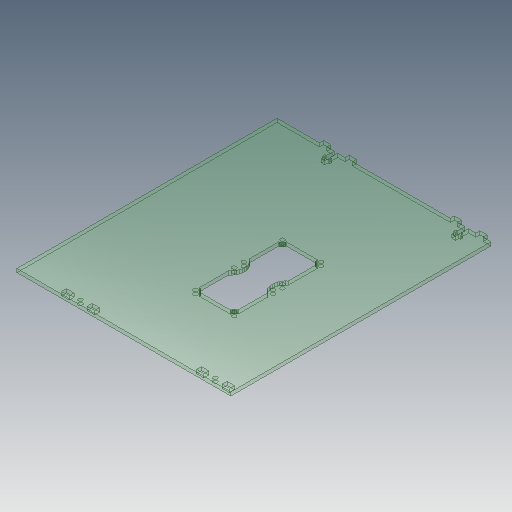
# Autodesk Inventor part: EE Top
Saved by Autodesk Inventor 2017 (Build 210142000, 142)
## iProperties
Created: 2016-07-27
Part Number: EE Top
Material: Polycarbonate, Green
Document SubType Name: Modeling
Designer: User
Density: 1.2 g/cm^3
Appearance: Polycarbonate - Clear(2)
Mass: 128.656 g
Surface Area: 752.573 cm^2
Volume: 107.213 cm^3
Author: User
Autodesk Inventor part; units mm, degrees
ref_plane "YZ Plane" through (0, 0, 0) normal (1, 0, 0) x (0, 1, 0)
ref_plane "XZ Plane" through (0, 0, 0) normal (0, 1, 0) x (-1, 0, 0)
ref_plane "XY Plane" through (0, 0, 0) normal (0, 0, 1) x (1, 0, 0)
sketch "Sketch1" plane through (0, 0, 0) normal (0, 1, 0) x (-1, 0, 0)
  line L0 (19.376, -30.1615) -> (19.376, -245.3788)
  line L1 (19.376, -245.3788) -> (25.876, -245.3788)
  line L2 (25.876, -245.3788) -> (25.876, -248.7288)
  line L3 (25.876, -248.7288) -> (31.8761, -248.7288)
  line L4 (31.8761, -248.7288) -> (31.8761, -245.3788)
  line L5 (31.8761, -245.3788) -> (37.9761, -245.3788)
  line L6 (37.9761, -245.3788) -> (37.9761, -239.3788)
  line L7 (37.9761, -239.3788) -> (36.7261, -239.3788)
  line L8 (36.7261, -239.3788) -> (36.7261, -237.3788)
  line L9 (36.7261, -237.3788) -> (37.9761, -237.3788)
  line L10 (37.9761, -237.3788) -> (37.9761, -234.7288)
  line L11 (37.9761, -234.7288) -> (40.9761, -234.7288)
  line L12 (40.9761, -234.7288) -> (40.9761, -237.3788)
  line L13 (40.9761, -237.3788) -> (42.226, -237.3788)
  line L14 (42.226, -237.3788) -> (42.226, -239.3788)
  line L15 (42.226, -239.3788) -> (40.9761, -239.3788)
  line L16 (40.9761, -239.3788) -> (40.9761, -245.3788)
  line L17 (40.9761, -245.3788) -> (47.0761, -245.3788)
  line L18 (47.0761, -245.3788) -> (47.0761, -248.7288)
  line L19 (47.0761, -248.7288) -> (53.076, -248.7288)
  line L20 (53.076, -248.7288) -> (53.076, -245.3788)
  line L21 (53.076, -245.3788) -> (53.1761, -245.3788)
  line L22 (53.1761, -245.3788) -> (134.0761, -245.3788)
  line L23 (134.0761, -245.3788) -> (134.0761, -248.7288)
  line L24 (134.0761, -248.7288) -> (140.0761, -248.7288)
  line L25 (140.0761, -248.7288) -> (140.0761, -245.3788)
  line L26 (140.0761, -245.3788) -> (146.176, -245.3788)
  line L27 (146.176, -245.3788) -> (146.176, -239.3788)
  line L28 (146.176, -239.3788) -> (144.926, -239.3788)
  line L29 (144.926, -239.3788) -> (144.926, -237.3788)
  line L30 (144.926, -237.3788) -> (146.176, -237.3788)
  line L31 (146.176, -237.3788) -> (146.176, -234.7288)
  line L32 (146.176, -234.7288) -> (149.1761, -234.7288)
  line L33 (149.1761, -234.7288) -> (149.1761, -237.3788)
  line L34 (149.1761, -237.3788) -> (150.4261, -237.3788)
  line L35 (150.4261, -237.3788) -> (150.4261, -239.3788)
  line L36 (150.4261, -239.3788) -> (149.1761, -239.3788)
  line L37 (149.1761, -239.3788) -> (149.1761, -245.3788)
  line L38 (149.1761, -245.3788) -> (155.2761, -245.3788)
  line L39 (155.2761, -245.3788) -> (155.2761, -248.7288)
  line L40 (155.2761, -248.7288) -> (161.276, -248.7288)
  line L41 (161.276, -248.7288) -> (161.276, -245.3788)
  line L42 (161.276, -245.3788) -> (161.376, -245.3788)
  line L43 (161.376, -245.3788) -> (196.376, -245.3788)
  line L44 (196.376, -245.3788) -> (196.376, -30.1615)
  line L45 (196.376, -30.1615) -> (19.376, -30.1615)
  line L46 (76.7649, -160.1938) -> (76.5951, -159.7839)
  line L47 (76.5951, -159.7839) -> (76.325, -159.4319)
  line L48 (76.325, -159.4319) -> (75.9729, -159.1617)
  line L49 (75.9729, -159.1617) -> (75.5628, -158.9919)
  line L50 (75.5628, -158.9919) -> (75.1229, -158.9339)
  line L51 (75.1229, -158.9339) -> (74.6829, -158.9919)
  line L52 (74.6829, -158.9919) -> (74.2729, -159.1617)
  line L53 (74.2729, -159.1617) -> (73.9208, -159.4319)
  line L54 (73.9208, -159.4319) -> (73.6506, -159.784)
  line L55 (73.6506, -159.784) -> (73.4808, -160.194)
  line L56 (73.4808, -160.194) -> (73.4229, -160.634)
  line L57 (73.4229, -160.634) -> (73.4808, -161.074)
  line L58 (73.4808, -161.074) -> (73.6506, -161.484)
  line L59 (73.6506, -161.484) -> (73.9208, -161.836)
  line L60 (73.9208, -161.836) -> (74.2729, -162.1062)
  line L61 (74.2729, -162.1062) -> (74.6829, -162.276)
  line L62 (74.6829, -162.276) -> (75.1229, -162.334)
  line L63 (75.1229, -162.334) -> (75.5629, -162.276)
  line L64 (75.5629, -162.276) -> (75.9729, -162.1062)
  line L65 (75.9729, -162.1062) -> (76.325, -161.836)
  line L66 (76.325, -161.836) -> (76.5951, -161.4839)
  line L67 (76.5951, -161.4839) -> (76.7649, -161.074)
  line L68 (76.7649, -161.074) -> (76.8229, -160.6339)
  line L69 (76.8229, -160.6339) -> (76.7649, -160.1938)
  line L70 (76.7642, -120.194) -> (76.5944, -119.784)
  line L71 (76.5944, -119.784) -> (76.3242, -119.4319)
  line L72 (76.3242, -119.4319) -> (75.9721, -119.1618)
  line L73 (75.9721, -119.1618) -> (75.5621, -118.992)
  line L74 (75.5621, -118.992) -> (75.1221, -118.934)
  line L75 (75.1221, -118.934) -> (74.6821, -118.992)
  line L76 (74.6821, -118.992) -> (74.2721, -119.1618)
  line L77 (74.2721, -119.1618) -> (73.9201, -119.4319)
  line L78 (73.9201, -119.4319) -> (73.6499, -119.7841)
  line L79 (73.6499, -119.7841) -> (73.48, -120.1941)
  line L80 (73.48, -120.1941) -> (73.4221, -120.6341)
  line L81 (73.4221, -120.6341) -> (73.48, -121.0741)
  line L82 (73.48, -121.0741) -> (73.6499, -121.4841)
  line L83 (73.6499, -121.4841) -> (73.92, -121.8361)
  line L84 (73.92, -121.8361) -> (74.2722, -122.1063)
  line L85 (74.2722, -122.1063) -> (74.6822, -122.2761)
  line L86 (74.6822, -122.2761) -> (75.1221, -122.3341)
  line L87 (75.1221, -122.3341) -> (75.5621, -122.2761)
  line L88 (75.5621, -122.2761) -> (75.9721, -122.1063)
  line L89 (75.9721, -122.1063) -> (76.3242, -121.8361)
  line L90 (76.3242, -121.8361) -> (76.5944, -121.484)
  line L91 (76.5944, -121.484) -> (76.7642, -121.074)
  line L92 (76.7642, -121.074) -> (76.8221, -120.634)
  line L93 (76.8221, -120.634) -> (76.7642, -120.194)
  line L94 (76.7643, -128.194) -> (76.5945, -127.784)
  line L95 (76.5945, -127.784) -> (76.3243, -127.4319)
  line L96 (76.3243, -127.4319) -> (75.9722, -127.1618)
  line L97 (75.9722, -127.1618) -> (75.5622, -126.9919)
  line L98 (75.5622, -126.9919) -> (75.1222, -126.934)
  line L99 (75.1222, -126.934) -> (74.6823, -126.992)
  line L100 (74.6823, -126.992) -> (74.2723, -127.1618)
  line L101 (74.2723, -127.1618) -> (73.9202, -127.432)
  line L102 (73.9202, -127.432) -> (73.65, -127.784)
  line L103 (73.65, -127.784) -> (73.4802, -128.194)
  line L104 (73.4802, -128.194) -> (73.4223, -128.6341)
  line L105 (73.4223, -128.6341) -> (73.4802, -129.074)
  line L106 (73.4802, -129.074) -> (73.65, -129.484)
  line L107 (73.65, -129.484) -> (73.9202, -129.8361)
  line L108 (73.9202, -129.8361) -> (74.2723, -130.1063)
  line L109 (74.2723, -130.1063) -> (74.6823, -130.2761)
  line L110 (74.6823, -130.2761) -> (75.1223, -130.3341)
  line L111 (75.1223, -130.3341) -> (75.5623, -130.2761)
  line L112 (75.5623, -130.2761) -> (75.9723, -130.1063)
  line L113 (75.9723, -130.1063) -> (76.3244, -129.8361)
  line L114 (76.3244, -129.8361) -> (76.5945, -129.484)
  line L115 (76.5945, -129.484) -> (76.7644, -129.074)
  line L116 (76.7644, -129.074) -> (76.8223, -128.6342)
  line L117 (76.8223, -128.6342) -> (76.7643, -128.194)
  line L118 (108.7657, -128.194) -> (108.5958, -127.7838)
  line L119 (108.5958, -127.7838) -> (108.3256, -127.4318)
  line L120 (108.3256, -127.4318) -> (107.9736, -127.1616)
  line L121 (107.9736, -127.1616) -> (107.5636, -126.9918)
  line L122 (107.5636, -126.9918) -> (107.1236, -126.9339)
  line L123 (107.1236, -126.9339) -> (106.6835, -126.9918)
  line L124 (106.6835, -126.9918) -> (106.2736, -127.1616)
  line L125 (106.2736, -127.1616) -> (105.9215, -127.4318)
  line L126 (105.9215, -127.4318) -> (105.6514, -127.7839)
  line L127 (105.6514, -127.7839) -> (105.4815, -128.1939)
  line L128 (105.4815, -128.1939) -> (105.4236, -128.6339)
  line L129 (105.4236, -128.6339) -> (105.4815, -129.0739)
  line L130 (105.4815, -129.0739) -> (105.6514, -129.4839)
  line L131 (105.6514, -129.4839) -> (105.9215, -129.8359)
  line L132 (105.9215, -129.8359) -> (106.2736, -130.1061)
  line L133 (106.2736, -130.1061) -> (106.6836, -130.2759)
  line L134 (106.6836, -130.2759) -> (107.1236, -130.3339)
  line L135 (107.1236, -130.3339) -> (107.5636, -130.2759)
  line L136 (107.5636, -130.2759) -> (107.9736, -130.1061)
  line L137 (107.9736, -130.1061) -> (108.3257, -129.8359)
  line L138 (108.3257, -129.8359) -> (108.5958, -129.4838)
  line L139 (108.5958, -129.4838) -> (108.7657, -129.0738)
  line L140 (108.7657, -129.0738) -> (108.8236, -128.6339)
  line L141 (108.8236, -128.6339) -> (108.7657, -128.194)
  line L142 (108.7648, -120.1938) -> (108.5951, -119.784)
  line L143 (108.5951, -119.784) -> (108.3249, -119.4319)
  line L144 (108.3249, -119.4319) -> (107.9728, -119.1617)
  line L145 (107.9728, -119.1617) -> (107.5628, -118.9919)
  line L146 (107.5628, -118.9919) -> (107.1228, -118.934)
  line L147 (107.1228, -118.934) -> (106.6828, -118.9919)
  line L148 (106.6828, -118.9919) -> (106.2728, -119.1617)
  line L149 (106.2728, -119.1617) -> (105.9207, -119.4319)
  line L150 (105.9207, -119.4319) -> (105.6506, -119.784)
  line L151 (105.6506, -119.784) -> (105.4807, -120.194)
  line L152 (105.4807, -120.194) -> (105.4228, -120.634)
  line L153 (105.4228, -120.634) -> (105.4808, -121.074)
  line L154 (105.4808, -121.074) -> (105.6506, -121.484)
  line L155 (105.6506, -121.484) -> (105.9208, -121.8361)
  line L156 (105.9208, -121.8361) -> (106.2728, -122.1062)
  line L157 (106.2728, -122.1062) -> (106.6828, -122.276)
  line L158 (106.6828, -122.276) -> (107.1229, -122.334)
  line L159 (107.1229, -122.334) -> (107.5628, -122.276)
  line L160 (107.5628, -122.276) -> (107.9728, -122.1062)
  line L161 (107.9728, -122.1062) -> (108.3249, -121.836)
  line L162 (108.3249, -121.836) -> (108.5951, -121.484)
  line L163 (108.5951, -121.484) -> (108.7649, -121.0739)
  line L164 (108.7649, -121.0739) -> (108.8228, -120.6341)
  line L165 (108.8228, -120.6341) -> (108.7648, -120.1938)
  line L166 (108.7648, -160.1937) -> (108.5951, -159.784)
  line L167 (108.5951, -159.784) -> (108.3249, -159.4319)
  line L168 (108.3249, -159.4319) -> (107.9728, -159.1617)
  line L169 (107.9728, -159.1617) -> (107.5628, -158.9919)
  line L170 (107.5628, -158.9919) -> (107.1228, -158.934)
  line L171 (107.1228, -158.934) -> (106.6828, -158.9919)
  line L172 (106.6828, -158.9919) -> (106.2728, -159.1617)
  line L173 (106.2728, -159.1617) -> (105.9207, -159.4319)
  line L174 (105.9207, -159.4319) -> (105.6506, -159.784)
  line L175 (105.6506, -159.784) -> (105.4807, -160.194)
  line L176 (105.4807, -160.194) -> (105.4228, -160.634)
  line L177 (105.4228, -160.634) -> (105.4808, -161.074)
  line L178 (105.4808, -161.074) -> (105.6506, -161.484)
  line L179 (105.6506, -161.484) -> (105.9208, -161.8361)
  line L180 (105.9208, -161.8361) -> (106.2728, -162.1062)
  line L181 (106.2728, -162.1062) -> (106.6828, -162.276)
  line L182 (106.6828, -162.276) -> (107.1228, -162.334)
  line L183 (107.1228, -162.334) -> (107.5628, -162.276)
  line L184 (107.5628, -162.276) -> (107.9728, -162.1062)
  line L185 (107.9728, -162.1062) -> (108.3249, -161.836)
  line L186 (108.3249, -161.836) -> (108.595, -161.4839)
  line L187 (108.595, -161.4839) -> (108.7649, -161.0739)
  line L188 (108.7649, -161.0739) -> (108.8228, -160.6341)
  line L189 (108.8228, -160.6341) -> (108.7648, -160.1937)
  line L190 (149.2477, -33.6616) -> (149.1238, -33.2802)
  line L191 (149.1238, -33.2802) -> (148.9088, -32.9416)
  line L192 (148.9088, -32.9416) -> (148.6165, -32.667)
  line L193 (148.6165, -32.667) -> (148.2651, -32.4738)
  line L194 (148.2651, -32.4738) -> (147.8766, -32.3741)
  line L195 (147.8766, -32.3741) -> (147.4755, -32.3741)
  line L196 (147.4755, -32.3741) -> (147.087, -32.4738)
  line L197 (147.087, -32.4738) -> (146.7356, -32.667)
  line L198 (146.7356, -32.667) -> (146.4432, -32.9416)
  line L199 (146.4432, -32.9416) -> (146.2283, -33.2802)
  line L200 (146.2283, -33.2802) -> (146.1044, -33.6616)
  line L201 (146.1044, -33.6616) -> (146.0792, -34.0619)
  line L202 (146.0792, -34.0619) -> (146.1543, -34.4559)
  line L203 (146.1543, -34.4559) -> (146.3251, -34.8188)
  line L204 (146.3251, -34.8188) -> (146.5807, -35.1278)
  line L205 (146.5807, -35.1278) -> (146.9052, -35.3635)
  line L206 (146.9052, -35.3635) -> (147.2781, -35.5112)
  line L207 (147.2781, -35.5112) -> (147.676, -35.5615)
  line L208 (147.676, -35.5615) -> (148.0739, -35.5112)
  line L209 (148.0739, -35.5112) -> (148.4468, -35.3636)
  line L210 (148.4468, -35.3636) -> (148.7713, -35.1278)
  line L211 (148.7713, -35.1278) -> (149.0269, -34.8188)
  line L212 (149.0269, -34.8188) -> (149.1977, -34.4559)
  line L213 (149.1977, -34.4559) -> (149.2729, -34.0619)
  line L214 (149.2729, -34.0619) -> (149.2477, -33.6616)
  line L215 (155.176, -32.0615) -> (155.176, -36.1614)
  line L216 (155.176, -36.1614) -> (161.376, -36.1614)
  line L217 (161.376, -36.1614) -> (161.376, -32.0615)
  line L218 (161.376, -32.0615) -> (155.176, -32.0615)
  line L219 (37.6477, -33.6616) -> (37.5238, -33.2802)
  line L220 (37.5238, -33.2802) -> (37.3089, -32.9416)
  line L221 (37.3089, -32.9416) -> (37.0165, -32.667)
  line L222 (37.0165, -32.667) -> (36.6651, -32.4738)
  line L223 (36.6651, -32.4738) -> (36.2766, -32.3741)
  line L224 (36.2766, -32.3741) -> (35.8755, -32.3741)
  line L225 (35.8755, -32.3741) -> (35.487, -32.4738)
  line L226 (35.487, -32.4738) -> (35.1356, -32.667)
  line L227 (35.1356, -32.667) -> (34.8432, -32.9416)
  line L228 (34.8432, -32.9416) -> (34.6283, -33.2802)
  line L229 (34.6283, -33.2802) -> (34.5044, -33.6616)
  line L230 (34.5044, -33.6616) -> (34.4792, -34.0619)
  line L231 (34.4792, -34.0619) -> (34.5543, -34.4559)
  line L232 (34.5543, -34.4559) -> (34.7251, -34.8188)
  line L233 (34.7251, -34.8188) -> (34.9808, -35.1278)
  line L234 (34.9808, -35.1278) -> (35.3052, -35.3636)
  line L235 (35.3052, -35.3636) -> (35.6781, -35.5112)
  line L236 (35.6781, -35.5112) -> (36.076, -35.5615)
  line L237 (36.076, -35.5615) -> (36.4739, -35.5112)
  line L238 (36.4739, -35.5112) -> (36.8469, -35.3636)
  line L239 (36.8469, -35.3636) -> (37.1713, -35.1278)
  line L240 (37.1713, -35.1278) -> (37.427, -34.8188)
  line L241 (37.427, -34.8188) -> (37.5977, -34.4559)
  line L242 (37.5977, -34.4559) -> (37.6729, -34.0619)
  line L243 (37.6729, -34.0619) -> (37.6477, -33.6616)
  line L244 (22.376, -32.0615) -> (22.376, -36.1614)
  line L245 (22.376, -36.1614) -> (28.576, -36.1614)
  line L246 (28.576, -36.1614) -> (28.576, -32.0615)
  line L247 (28.576, -32.0615) -> (22.376, -32.0615)
  line L248 (76.7631, -88.1941) -> (76.5933, -87.7842)
  line L249 (76.5933, -87.7842) -> (76.3232, -87.4321)
  line L250 (76.3232, -87.4321) -> (75.9711, -87.162)
  line L251 (75.9711, -87.162) -> (75.5611, -86.9921)
  line L252 (75.5611, -86.9921) -> (75.1211, -86.9342)
  line L253 (75.1211, -86.9342) -> (74.6811, -86.9921)
  line L254 (74.6811, -86.9921) -> (74.2711, -87.162)
  line L255 (74.2711, -87.162) -> (73.919, -87.4321)
  line L256 (73.919, -87.4321) -> (73.6489, -87.7842)
  line L257 (73.6489, -87.7842) -> (73.479, -88.1942)
  line L258 (73.479, -88.1942) -> (73.4211, -88.6342)
  line L259 (73.4211, -88.6342) -> (73.479, -89.0742)
  line L260 (73.479, -89.0742) -> (73.6489, -89.4842)
  line L261 (73.6489, -89.4842) -> (73.919, -89.8363)
  line L262 (73.919, -89.8363) -> (74.2711, -90.1064)
  line L263 (74.2711, -90.1064) -> (74.6811, -90.2763)
  line L264 (74.6811, -90.2763) -> (75.1211, -90.3342)
  line L265 (75.1211, -90.3342) -> (75.5611, -90.2763)
  line L266 (75.5611, -90.2763) -> (75.9711, -90.1064)
  line L267 (75.9711, -90.1064) -> (76.3232, -89.8363)
  line L268 (76.3232, -89.8363) -> (76.5933, -89.4842)
  line L269 (76.5933, -89.4842) -> (76.7632, -89.0742)
  line L270 (76.7632, -89.0742) -> (76.8211, -88.6342)
  line L271 (76.8211, -88.6342) -> (76.7631, -88.1941)
  line L272 (43.576, -32.0615) -> (43.576, -36.1614)
  line L273 (43.576, -36.1614) -> (49.7761, -36.1614)
  line L274 (49.7761, -36.1614) -> (49.7761, -32.0615)
  line L275 (49.7761, -32.0615) -> (43.576, -32.0615)
  line L276 (103.3316, -121.3347) -> (103.9565, -119.7817)
  line L277 (103.9565, -119.7817) -> (104.8108, -118.342)
  line L278 (104.8108, -118.342) -> (105.8745, -117.0494)
  line L279 (105.8745, -117.0494) -> (107.1228, -115.934)
  line L280 (107.1228, -115.934) -> (107.1228, -91.834)
  line L281 (107.1228, -91.834) -> (106.7272, -91.7535)
  line L282 (106.7272, -91.7535) -> (106.3423, -91.6314)
  line L283 (106.3423, -91.6314) -> (105.9725, -91.4692)
  line L284 (105.9725, -91.4692) -> (105.622, -91.2688)
  line L285 (105.622, -91.2688) -> (105.2948, -91.0322)
  line L286 (105.2948, -91.0322) -> (104.9946, -90.7622)
  line L287 (104.9946, -90.7622) -> (104.7246, -90.462)
  line L288 (104.7246, -90.462) -> (104.488, -90.1347)
  line L289 (104.488, -90.1347) -> (104.2876, -89.7843)
  line L290 (104.2876, -89.7843) -> (104.1254, -89.4145)
  line L291 (104.1254, -89.4145) -> (104.0033, -89.0296)
  line L292 (104.0033, -89.0296) -> (103.9228, -88.634)
  line L293 (103.9228, -88.634) -> (78.3228, -88.634)
  line L294 (78.3228, -88.634) -> (78.2515, -89.0338)
  line L295 (78.2515, -89.0338) -> (78.1364, -89.4233)
  line L296 (78.1364, -89.4233) -> (77.979, -89.7977)
  line L297 (77.979, -89.7977) -> (77.7813, -90.1524)
  line L298 (77.7813, -90.1524) -> (77.5455, -90.4832)
  line L299 (77.5455, -90.4832) -> (77.2746, -90.7858)
  line L300 (77.2746, -90.7858) -> (76.972, -91.0566)
  line L301 (76.972, -91.0566) -> (76.6413, -91.2924)
  line L302 (76.6413, -91.2924) -> (76.2866, -91.4902)
  line L303 (76.2866, -91.4902) -> (75.9122, -91.6476)
  line L304 (75.9122, -91.6476) -> (75.5227, -91.7626)
  line L305 (75.5227, -91.7626) -> (75.1228, -91.834)
  line L306 (75.1228, -91.834) -> (75.1228, -115.934)
  line L307 (75.1228, -115.934) -> (76.3711, -117.0494)
  line L308 (76.3711, -117.0494) -> (77.4349, -118.342)
  line L309 (77.4349, -118.342) -> (78.2891, -119.7817)
  line L310 (78.2891, -119.7817) -> (78.914, -121.3347)
  line L311 (78.914, -121.3347) -> (79.2949, -122.9648)
  line L312 (79.2949, -122.9648) -> (79.4228, -124.634)
  line L313 (79.4228, -124.634) -> (79.2949, -126.3031)
  line L314 (79.2949, -126.3031) -> (78.914, -127.9333)
  line L315 (78.914, -127.9333) -> (78.2891, -129.4863)
  line L316 (78.2891, -129.4863) -> (77.4349, -130.9259)
  line L317 (77.4349, -130.9259) -> (76.3711, -132.2186)
  line L318 (76.3711, -132.2186) -> (75.1228, -133.334)
  line L319 (75.1228, -133.334) -> (75.1228, -157.434)
  line L320 (75.1228, -157.434) -> (75.5524, -157.4264)
  line L321 (75.5524, -157.4264) -> (75.9786, -157.4813)
  line L322 (75.9786, -157.4813) -> (76.3922, -157.5977)
  line L323 (76.3922, -157.5977) -> (76.7845, -157.7731)
  line L324 (76.7845, -157.7731) -> (77.1471, -158.0036)
  line L325 (77.1471, -158.0036) -> (77.4723, -158.2845)
  line L326 (77.4723, -158.2845) -> (77.7532, -158.6097)
  line L327 (77.7532, -158.6097) -> (77.9837, -158.9723)
  line L328 (77.9837, -158.9723) -> (78.1591, -159.3646)
  line L329 (78.1591, -159.3646) -> (78.2755, -159.7782)
  line L330 (78.2755, -159.7782) -> (78.3304, -160.2043)
  line L331 (78.3304, -160.2043) -> (78.3228, -160.634)
  line L332 (78.3228, -160.634) -> (103.9228, -160.634)
  line L333 (103.9228, -160.634) -> (104.0073, -160.2402)
  line L334 (104.0073, -160.2402) -> (104.1324, -159.8573)
  line L335 (104.1324, -159.8573) -> (104.2966, -159.4896)
  line L336 (104.2966, -159.4896) -> (104.4983, -159.1409)
  line L337 (104.4983, -159.1409) -> (104.7352, -158.8152)
  line L338 (104.7352, -158.8152) -> (105.0048, -158.516)
  line L339 (105.0048, -158.516) -> (105.3041, -158.2464)
  line L340 (105.3041, -158.2464) -> (105.6298, -158.0095)
  line L341 (105.6298, -158.0095) -> (105.9784, -157.8078)
  line L342 (105.9784, -157.8078) -> (106.3462, -157.6435)
  line L343 (106.3462, -157.6435) -> (106.729, -157.5185)
  line L344 (106.729, -157.5185) -> (107.1228, -157.434)
  line L345 (107.1228, -157.434) -> (107.1228, -133.334)
  line L346 (107.1228, -133.334) -> (105.8745, -132.2186)
  line L347 (105.8745, -132.2186) -> (104.8108, -130.9259)
  line L348 (104.8108, -130.9259) -> (103.9565, -129.4863)
  line L349 (103.9565, -129.4863) -> (103.3316, -127.9333)
  line L350 (103.3316, -127.9333) -> (102.9508, -126.3031)
  line L351 (102.9508, -126.3031) -> (102.8228, -124.634)
  line L352 (102.8228, -124.634) -> (102.9508, -122.9648)
  line L353 (102.9508, -122.9648) -> (103.3316, -121.3347)
  line L354 (108.7664, -88.1938) -> (108.5965, -87.7838)
  line L355 (108.5965, -87.7838) -> (108.3264, -87.4317)
  line L356 (108.3264, -87.4317) -> (107.9743, -87.1615)
  line L357 (107.9743, -87.1615) -> (107.5643, -86.9917)
  line L358 (107.5643, -86.9917) -> (107.1243, -86.9338)
  line L359 (107.1243, -86.9338) -> (106.6843, -86.9917)
  line L360 (106.6843, -86.9917) -> (106.2743, -87.1616)
  line L361 (106.2743, -87.1616) -> (105.9222, -87.4317)
  line L362 (105.9222, -87.4317) -> (105.6521, -87.7838)
  line L363 (105.6521, -87.7838) -> (105.4823, -88.1938)
  line L364 (105.4823, -88.1938) -> (105.4243, -88.6338)
  line L365 (105.4243, -88.6338) -> (105.4823, -89.0738)
  line L366 (105.4823, -89.0738) -> (105.6521, -89.4838)
  line L367 (105.6521, -89.4838) -> (105.9223, -89.8359)
  line L368 (105.9223, -89.8359) -> (106.2744, -90.106)
  line L369 (106.2744, -90.106) -> (106.6843, -90.2758)
  line L370 (106.6843, -90.2758) -> (107.1244, -90.3338)
  line L371 (107.1244, -90.3338) -> (107.5643, -90.2758)
  line L372 (107.5643, -90.2758) -> (107.9743, -90.106)
  line L373 (107.9743, -90.106) -> (108.3264, -89.8358)
  line L374 (108.3264, -89.8358) -> (108.5965, -89.4838)
  line L375 (108.5965, -89.4838) -> (108.7664, -89.0738)
  line L376 (108.7664, -89.0738) -> (108.8243, -88.6336)
  line L377 (108.8243, -88.6336) -> (108.7664, -88.1938)
  line L378 (133.976, -32.0615) -> (133.976, -36.1614)
  line L379 (133.976, -36.1614) -> (140.176, -36.1614)
  line L380 (140.176, -36.1614) -> (140.176, -32.0615)
  line L381 (140.176, -32.0615) -> (133.976, -32.0615)
  constraints: 764 end point, 181 parallel, 106 perpendicular, 3 collinear
extrude "Extrusion1" add sketch "Sketch1" along normal blind 3
sketch "Sketch2" plane through (0, 3, 0) normal (0, 1, 0) x (1, 0, 0)
  line L0 (-103.3316, 121.3347) -> (-102.9508, 122.9648) projected
  line L1 (-102.9508, 122.9648) -> (-102.8228, 124.634) projected
  line L2 (-102.8228, 124.634) -> (-102.9508, 126.3031) projected
  line L3 (-102.9508, 126.3031) -> (-103.3316, 127.9333) projected
  line L4 (-103.3316, 127.9333) -> (-103.9565, 129.4863) projected
  line L5 (-103.9565, 129.4863) -> (-104.8108, 130.9259) projected
  line L6 (-104.8108, 130.9259) -> (-105.8745, 132.2186) projected
  line L7 (-105.8745, 132.2186) -> (-107.1228, 133.334) projected
  line L8 (-107.1228, 133.334) -> (-107.1228, 157.434) projected
  line L9 (-107.1228, 157.434) -> (-106.729, 157.5185) projected
  line L10 (-106.729, 157.5185) -> (-106.3462, 157.6435) projected
  line L11 (-106.3462, 157.6435) -> (-105.9784, 157.8078) projected
  line L12 (-105.9784, 157.8078) -> (-105.6298, 158.0095) projected
  line L13 (-105.6298, 158.0095) -> (-105.3041, 158.2464) projected
  line L14 (-105.3041, 158.2464) -> (-105.0048, 158.516) projected
  line L15 (-105.0048, 158.516) -> (-104.7352, 158.8152) projected
  line L16 (-104.7352, 158.8152) -> (-104.4983, 159.1409) projected
  line L17 (-104.4983, 159.1409) -> (-104.2966, 159.4896) projected
  line L18 (-104.2966, 159.4896) -> (-104.1324, 159.8573) projected
  line L19 (-104.1324, 159.8573) -> (-104.0073, 160.2402) projected
  line L20 (-104.0073, 160.2402) -> (-103.9228, 160.634) projected
  line L21 (-103.9228, 160.634) -> (-78.3228, 160.634) projected
  line L22 (-78.3228, 160.634) -> (-78.3304, 160.2043) projected
  line L23 (-78.3304, 160.2043) -> (-78.2755, 159.7782) projected
  line L24 (-78.2755, 159.7782) -> (-78.1591, 159.3646) projected
  line L25 (-78.1591, 159.3646) -> (-77.9837, 158.9723) projected
  line L26 (-77.9837, 158.9723) -> (-77.7532, 158.6097) projected
  line L27 (-77.7532, 158.6097) -> (-77.4723, 158.2845) projected
  line L28 (-77.4723, 158.2845) -> (-77.1471, 158.0036) projected
  line L29 (-77.1471, 158.0036) -> (-76.7845, 157.7731) projected
  line L30 (-76.7845, 157.7731) -> (-76.3922, 157.5977) projected
  line L31 (-76.3922, 157.5977) -> (-75.9786, 157.4813) projected
  line L32 (-75.9786, 157.4813) -> (-75.5524, 157.4264) projected
  line L33 (-75.5524, 157.4264) -> (-75.1228, 157.434) projected
  line L34 (-75.1228, 157.434) -> (-75.1228, 133.334) projected
  line L35 (-75.1228, 133.334) -> (-76.3711, 132.2186) projected
  line L36 (-76.3711, 132.2186) -> (-77.4349, 130.9259) projected
  line L37 (-77.4349, 130.9259) -> (-78.2891, 129.4863) projected
  line L38 (-78.2891, 129.4863) -> (-78.914, 127.9333) projected
  line L39 (-78.914, 127.9333) -> (-79.2949, 126.3031) projected
  line L40 (-79.2949, 126.3031) -> (-79.4228, 124.634) projected
  line L41 (-79.4228, 124.634) -> (-79.2949, 122.9648) projected
  line L42 (-79.2949, 122.9648) -> (-78.914, 121.3347) projected
  line L43 (-78.914, 121.3347) -> (-78.2891, 119.7817) projected
  line L44 (-78.2891, 119.7817) -> (-77.4349, 118.342) projected
  line L45 (-77.4349, 118.342) -> (-76.3711, 117.0494) projected
  line L46 (-76.3711, 117.0494) -> (-75.1228, 115.934) projected
  line L47 (-75.1228, 115.934) -> (-75.1228, 91.834) projected
  line L48 (-75.1228, 91.834) -> (-75.5227, 91.7626) projected
  line L49 (-75.5227, 91.7626) -> (-75.9122, 91.6476) projected
  line L50 (-75.9122, 91.6476) -> (-76.2866, 91.4902) projected
  line L51 (-76.2866, 91.4902) -> (-76.6413, 91.2924) projected
  line L52 (-76.6413, 91.2924) -> (-76.972, 91.0566) projected
  line L53 (-76.972, 91.0566) -> (-77.2746, 90.7858) projected
  line L54 (-77.2746, 90.7858) -> (-77.5455, 90.4832) projected
  line L55 (-77.5455, 90.4832) -> (-77.7813, 90.1524) projected
  line L56 (-77.7813, 90.1524) -> (-77.979, 89.7977) projected
  line L57 (-77.979, 89.7977) -> (-78.1364, 89.4233) projected
  line L58 (-78.1364, 89.4233) -> (-78.2515, 89.0338) projected
  line L59 (-78.2515, 89.0338) -> (-78.3228, 88.634) projected
  line L60 (-78.3228, 88.634) -> (-103.9228, 88.634) projected
  line L61 (-103.9228, 88.634) -> (-104.0033, 89.0296) projected
  line L62 (-104.0033, 89.0296) -> (-104.1254, 89.4145) projected
  line L63 (-104.1254, 89.4145) -> (-104.2876, 89.7843) projected
  line L64 (-104.2876, 89.7843) -> (-104.488, 90.1347) projected
  line L65 (-104.488, 90.1347) -> (-104.7246, 90.462) projected
  line L66 (-104.7246, 90.462) -> (-104.9946, 90.7622) projected
  line L67 (-104.9946, 90.7622) -> (-105.2948, 91.0322) projected
  line L68 (-105.2948, 91.0322) -> (-105.622, 91.2688) projected
  line L69 (-105.622, 91.2688) -> (-105.9725, 91.4692) projected
  line L70 (-105.9725, 91.4692) -> (-106.3423, 91.6314) projected
  line L71 (-106.3423, 91.6314) -> (-106.7272, 91.7535) projected
  line L72 (-106.7272, 91.7535) -> (-107.1228, 91.834) projected
  line L73 (-107.1228, 91.834) -> (-107.1228, 115.934) projected
  line L74 (-107.1228, 115.934) -> (-105.8745, 117.0494) projected
  line L75 (-105.8745, 117.0494) -> (-104.8108, 118.342) projected
  line L76 (-104.8108, 118.342) -> (-103.9565, 119.7817) projected
  line L77 (-103.9565, 119.7817) -> (-103.3316, 121.3347) projected
  line L78 (-155.176, 32.0615) -> (-161.376, 32.0615) projected
  line L79 (-161.376, 32.0615) -> (-161.376, 36.1614) projected
  line L80 (-161.376, 36.1614) -> (-155.176, 36.1614) projected
  line L81 (-155.176, 36.1614) -> (-155.176, 32.0615) projected
  line L82 (-43.576, 32.0615) -> (-49.7761, 32.0615) projected
  line L83 (-49.7761, 32.0615) -> (-49.7761, 36.1614) projected
  line L84 (-49.7761, 36.1614) -> (-43.576, 36.1614) projected
  line L85 (-43.576, 36.1614) -> (-43.576, 32.0615) projected
  line L86 (-133.976, 32.0615) -> (-140.176, 32.0615) projected
  line L87 (-140.176, 32.0615) -> (-140.176, 36.1614) projected
  line L88 (-140.176, 36.1614) -> (-133.976, 36.1614) projected
  line L89 (-133.976, 36.1614) -> (-133.976, 32.0615) projected
  line L90 (-22.376, 32.0615) -> (-28.576, 32.0615) projected
  line L91 (-28.576, 32.0615) -> (-28.576, 36.1614) projected
  line L92 (-28.576, 36.1614) -> (-22.376, 36.1614) projected
  line L93 (-22.376, 36.1614) -> (-22.376, 32.0615) projected
  line L94 (-76.7642, 120.194) -> (-76.8221, 120.634) projected
  line L95 (-76.8221, 120.634) -> (-76.7642, 121.074) projected
  line L96 (-76.7642, 121.074) -> (-76.5944, 121.484) projected
  line L97 (-76.5944, 121.484) -> (-76.3242, 121.8361) projected
  line L98 (-76.3242, 121.8361) -> (-75.9721, 122.1063) projected
  line L99 (-75.9721, 122.1063) -> (-75.5621, 122.2761) projected
  line L100 (-75.5621, 122.2761) -> (-75.1221, 122.3341) projected
  line L101 (-75.1221, 122.3341) -> (-74.6822, 122.2761) projected
  line L102 (-74.6822, 122.2761) -> (-74.2722, 122.1063) projected
  line L103 (-74.2722, 122.1063) -> (-73.92, 121.8361) projected
  line L104 (-73.92, 121.8361) -> (-73.6499, 121.4841) projected
  line L105 (-73.6499, 121.4841) -> (-73.48, 121.0741) projected
  line L106 (-73.48, 121.0741) -> (-73.4221, 120.6341) projected
  line L107 (-73.4221, 120.6341) -> (-73.48, 120.1941) projected
  line L108 (-73.48, 120.1941) -> (-73.6499, 119.7841) projected
  line L109 (-73.6499, 119.7841) -> (-73.9201, 119.4319) projected
  line L110 (-73.9201, 119.4319) -> (-74.2721, 119.1618) projected
  line L111 (-74.2721, 119.1618) -> (-74.6821, 118.992) projected
  line L112 (-74.6821, 118.992) -> (-75.1221, 118.934) projected
  line L113 (-75.1221, 118.934) -> (-75.5621, 118.992) projected
  line L114 (-75.5621, 118.992) -> (-75.9721, 119.1618) projected
  line L115 (-75.9721, 119.1618) -> (-76.3242, 119.4319) projected
  line L116 (-76.3242, 119.4319) -> (-76.5944, 119.784) projected
  line L117 (-76.5944, 119.784) -> (-76.7642, 120.194) projected
  line L118 (-76.7643, 128.194) -> (-76.8223, 128.6342) projected
  line L119 (-76.8223, 128.6342) -> (-76.7644, 129.074) projected
  line L120 (-76.7644, 129.074) -> (-76.5945, 129.484) projected
  line L121 (-76.5945, 129.484) -> (-76.3244, 129.8361) projected
  line L122 (-76.3244, 129.8361) -> (-75.9723, 130.1063) projected
  line L123 (-75.9723, 130.1063) -> (-75.5623, 130.2761) projected
  line L124 (-75.5623, 130.2761) -> (-75.1223, 130.3341) projected
  line L125 (-75.1223, 130.3341) -> (-74.6823, 130.2761) projected
  line L126 (-74.6823, 130.2761) -> (-74.2723, 130.1063) projected
  line L127 (-74.2723, 130.1063) -> (-73.9202, 129.8361) projected
  line L128 (-73.9202, 129.8361) -> (-73.65, 129.484) projected
  line L129 (-73.65, 129.484) -> (-73.4802, 129.074) projected
  line L130 (-73.4802, 129.074) -> (-73.4223, 128.6341) projected
  line L131 (-73.4223, 128.6341) -> (-73.4802, 128.194) projected
  line L132 (-73.4802, 128.194) -> (-73.65, 127.784) projected
  line L133 (-73.65, 127.784) -> (-73.9202, 127.432) projected
  line L134 (-73.9202, 127.432) -> (-74.2723, 127.1618) projected
  line L135 (-74.2723, 127.1618) -> (-74.6823, 126.992) projected
  line L136 (-74.6823, 126.992) -> (-75.1222, 126.934) projected
  line L137 (-75.1222, 126.934) -> (-75.5622, 126.9919) projected
  line L138 (-75.5622, 126.9919) -> (-75.9722, 127.1618) projected
  line L139 (-75.9722, 127.1618) -> (-76.3243, 127.4319) projected
  line L140 (-76.3243, 127.4319) -> (-76.5945, 127.784) projected
  line L141 (-76.5945, 127.784) -> (-76.7643, 128.194) projected
  line L142 (-76.7649, 160.1938) -> (-76.8229, 160.6339) projected
  line L143 (-76.8229, 160.6339) -> (-76.7649, 161.074) projected
  line L144 (-76.7649, 161.074) -> (-76.5951, 161.4839) projected
  line L145 (-76.5951, 161.4839) -> (-76.325, 161.836) projected
  line L146 (-76.325, 161.836) -> (-75.9729, 162.1062) projected
  line L147 (-75.9729, 162.1062) -> (-75.5629, 162.276) projected
  line L148 (-75.5629, 162.276) -> (-75.1229, 162.334) projected
  line L149 (-75.1229, 162.334) -> (-74.6829, 162.276) projected
  line L150 (-74.6829, 162.276) -> (-74.2729, 162.1062) projected
  line L151 (-74.2729, 162.1062) -> (-73.9208, 161.836) projected
  line L152 (-73.9208, 161.836) -> (-73.6506, 161.484) projected
  line L153 (-73.6506, 161.484) -> (-73.4808, 161.074) projected
  line L154 (-73.4808, 161.074) -> (-73.4229, 160.634) projected
  line L155 (-73.4229, 160.634) -> (-73.4808, 160.194) projected
  line L156 (-73.4808, 160.194) -> (-73.6506, 159.784) projected
  line L157 (-73.6506, 159.784) -> (-73.9208, 159.4319) projected
  line L158 (-73.9208, 159.4319) -> (-74.2729, 159.1617) projected
  line L159 (-74.2729, 159.1617) -> (-74.6829, 158.9919) projected
  line L160 (-74.6829, 158.9919) -> (-75.1229, 158.9339) projected
  line L161 (-75.1229, 158.9339) -> (-75.5628, 158.9919) projected
  line L162 (-75.5628, 158.9919) -> (-75.9729, 159.1617) projected
  line L163 (-75.9729, 159.1617) -> (-76.325, 159.4319) projected
  line L164 (-76.325, 159.4319) -> (-76.5951, 159.7839) projected
  line L165 (-76.5951, 159.7839) -> (-76.7649, 160.1938) projected
  line L166 (-76.7631, 88.1941) -> (-76.8211, 88.6342) projected
  line L167 (-76.8211, 88.6342) -> (-76.7632, 89.0742) projected
  line L168 (-76.7632, 89.0742) -> (-76.5933, 89.4842) projected
  line L169 (-76.5933, 89.4842) -> (-76.3232, 89.8363) projected
  line L170 (-76.3232, 89.8363) -> (-75.9711, 90.1064) projected
  line L171 (-75.9711, 90.1064) -> (-75.5611, 90.2763) projected
  line L172 (-75.5611, 90.2763) -> (-75.1211, 90.3342) projected
  line L173 (-75.1211, 90.3342) -> (-74.6811, 90.2763) projected
  line L174 (-74.6811, 90.2763) -> (-74.2711, 90.1064) projected
  line L175 (-74.2711, 90.1064) -> (-73.919, 89.8363) projected
  line L176 (-73.919, 89.8363) -> (-73.6489, 89.4842) projected
  line L177 (-73.6489, 89.4842) -> (-73.479, 89.0742) projected
  line L178 (-73.479, 89.0742) -> (-73.4211, 88.6342) projected
  line L179 (-73.4211, 88.6342) -> (-73.479, 88.1942) projected
  line L180 (-73.479, 88.1942) -> (-73.6489, 87.7842) projected
  line L181 (-73.6489, 87.7842) -> (-73.919, 87.4321) projected
  line L182 (-73.919, 87.4321) -> (-74.2711, 87.162) projected
  line L183 (-74.2711, 87.162) -> (-74.6811, 86.9921) projected
  line L184 (-74.6811, 86.9921) -> (-75.1211, 86.9342) projected
  line L185 (-75.1211, 86.9342) -> (-75.5611, 86.9921) projected
  line L186 (-75.5611, 86.9921) -> (-75.9711, 87.162) projected
  line L187 (-75.9711, 87.162) -> (-76.3232, 87.4321) projected
  line L188 (-76.3232, 87.4321) -> (-76.5933, 87.7842) projected
  line L189 (-76.5933, 87.7842) -> (-76.7631, 88.1941) projected
  line L190 (-108.7657, 128.194) -> (-108.8236, 128.6339) projected
  line L191 (-108.8236, 128.6339) -> (-108.7657, 129.0738) projected
  line L192 (-108.7657, 129.0738) -> (-108.5958, 129.4838) projected
  line L193 (-108.5958, 129.4838) -> (-108.3257, 129.8359) projected
  line L194 (-108.3257, 129.8359) -> (-107.9736, 130.1061) projected
  line L195 (-107.9736, 130.1061) -> (-107.5636, 130.2759) projected
  line L196 (-107.5636, 130.2759) -> (-107.1236, 130.3339) projected
  line L197 (-107.1236, 130.3339) -> (-106.6836, 130.2759) projected
  line L198 (-106.6836, 130.2759) -> (-106.2736, 130.1061) projected
  line L199 (-106.2736, 130.1061) -> (-105.9215, 129.8359) projected
  line L200 (-105.9215, 129.8359) -> (-105.6514, 129.4839) projected
  line L201 (-105.6514, 129.4839) -> (-105.4815, 129.0739) projected
  line L202 (-105.4815, 129.0739) -> (-105.4236, 128.6339) projected
  line L203 (-105.4236, 128.6339) -> (-105.4815, 128.1939) projected
  line L204 (-105.4815, 128.1939) -> (-105.6514, 127.7839) projected
  line L205 (-105.6514, 127.7839) -> (-105.9215, 127.4318) projected
  line L206 (-105.9215, 127.4318) -> (-106.2736, 127.1616) projected
  line L207 (-106.2736, 127.1616) -> (-106.6835, 126.9918) projected
  line L208 (-106.6835, 126.9918) -> (-107.1236, 126.9339) projected
  line L209 (-107.1236, 126.9339) -> (-107.5636, 126.9918) projected
  line L210 (-107.5636, 126.9918) -> (-107.9736, 127.1616) projected
  line L211 (-107.9736, 127.1616) -> (-108.3256, 127.4318) projected
  line L212 (-108.3256, 127.4318) -> (-108.5958, 127.7838) projected
  line L213 (-108.5958, 127.7838) -> (-108.7657, 128.194) projected
  line L214 (-108.7648, 120.1938) -> (-108.8228, 120.6341) projected
  line L215 (-108.8228, 120.6341) -> (-108.7649, 121.0739) projected
  line L216 (-108.7649, 121.0739) -> (-108.5951, 121.484) projected
  line L217 (-108.5951, 121.484) -> (-108.3249, 121.836) projected
  line L218 (-108.3249, 121.836) -> (-107.9728, 122.1062) projected
  line L219 (-107.9728, 122.1062) -> (-107.5628, 122.276) projected
  line L220 (-107.5628, 122.276) -> (-107.1229, 122.334) projected
  line L221 (-107.1229, 122.334) -> (-106.6828, 122.276) projected
  line L222 (-106.6828, 122.276) -> (-106.2728, 122.1062) projected
  line L223 (-106.2728, 122.1062) -> (-105.9208, 121.8361) projected
  line L224 (-105.9208, 121.8361) -> (-105.6506, 121.484) projected
  line L225 (-105.6506, 121.484) -> (-105.4808, 121.074) projected
  line L226 (-105.4808, 121.074) -> (-105.4228, 120.634) projected
  line L227 (-105.4228, 120.634) -> (-105.4807, 120.194) projected
  line L228 (-105.4807, 120.194) -> (-105.6506, 119.784) projected
  line L229 (-105.6506, 119.784) -> (-105.9207, 119.4319) projected
  line L230 (-105.9207, 119.4319) -> (-106.2728, 119.1617) projected
  line L231 (-106.2728, 119.1617) -> (-106.6828, 118.9919) projected
  line L232 (-106.6828, 118.9919) -> (-107.1228, 118.934) projected
  line L233 (-107.1228, 118.934) -> (-107.5628, 118.9919) projected
  line L234 (-107.5628, 118.9919) -> (-107.9728, 119.1617) projected
  line L235 (-107.9728, 119.1617) -> (-108.3249, 119.4319) projected
  line L236 (-108.3249, 119.4319) -> (-108.5951, 119.784) projected
  line L237 (-108.5951, 119.784) -> (-108.7648, 120.1938) projected
  line L238 (-108.7648, 160.1937) -> (-108.8228, 160.6341) projected
  line L239 (-108.8228, 160.6341) -> (-108.7649, 161.0739) projected
  line L240 (-108.7649, 161.0739) -> (-108.595, 161.4839) projected
  line L241 (-108.595, 161.4839) -> (-108.3249, 161.836) projected
  line L242 (-108.3249, 161.836) -> (-107.9728, 162.1062) projected
  line L243 (-107.9728, 162.1062) -> (-107.5628, 162.276) projected
  line L244 (-107.5628, 162.276) -> (-107.1228, 162.334) projected
  line L245 (-107.1228, 162.334) -> (-106.6828, 162.276) projected
  line L246 (-106.6828, 162.276) -> (-106.2728, 162.1062) projected
  line L247 (-106.2728, 162.1062) -> (-105.9208, 161.8361) projected
  line L248 (-105.9208, 161.8361) -> (-105.6506, 161.484) projected
  line L249 (-105.6506, 161.484) -> (-105.4808, 161.074) projected
  line L250 (-105.4808, 161.074) -> (-105.4228, 160.634) projected
  line L251 (-105.4228, 160.634) -> (-105.4807, 160.194) projected
  line L252 (-105.4807, 160.194) -> (-105.6506, 159.784) projected
  line L253 (-105.6506, 159.784) -> (-105.9207, 159.4319) projected
  line L254 (-105.9207, 159.4319) -> (-106.2728, 159.1617) projected
  line L255 (-106.2728, 159.1617) -> (-106.6828, 158.9919) projected
  line L256 (-106.6828, 158.9919) -> (-107.1228, 158.934) projected
  line L257 (-107.1228, 158.934) -> (-107.5628, 158.9919) projected
  line L258 (-107.5628, 158.9919) -> (-107.9728, 159.1617) projected
  line L259 (-107.9728, 159.1617) -> (-108.3249, 159.4319) projected
  line L260 (-108.3249, 159.4319) -> (-108.5951, 159.784) projected
  line L261 (-108.5951, 159.784) -> (-108.7648, 160.1937) projected
  line L262 (-108.7664, 88.1938) -> (-108.8243, 88.6336) projected
  line L263 (-108.8243, 88.6336) -> (-108.7664, 89.0738) projected
  line L264 (-108.7664, 89.0738) -> (-108.5965, 89.4838) projected
  line L265 (-108.5965, 89.4838) -> (-108.3264, 89.8358) projected
  line L266 (-108.3264, 89.8358) -> (-107.9743, 90.106) projected
  line L267 (-107.9743, 90.106) -> (-107.5643, 90.2758) projected
  line L268 (-107.5643, 90.2758) -> (-107.1244, 90.3338) projected
  line L269 (-107.1244, 90.3338) -> (-106.6843, 90.2758) projected
  line L270 (-106.6843, 90.2758) -> (-106.2744, 90.106) projected
  line L271 (-106.2744, 90.106) -> (-105.9223, 89.8359) projected
  line L272 (-105.9223, 89.8359) -> (-105.6521, 89.4838) projected
  line L273 (-105.6521, 89.4838) -> (-105.4823, 89.0738) projected
  line L274 (-105.4823, 89.0738) -> (-105.4243, 88.6338) projected
  line L275 (-105.4243, 88.6338) -> (-105.4823, 88.1938) projected
  line L276 (-105.4823, 88.1938) -> (-105.6521, 87.7838) projected
  line L277 (-105.6521, 87.7838) -> (-105.9222, 87.4317) projected
  line L278 (-105.9222, 87.4317) -> (-106.2743, 87.1616) projected
  line L279 (-106.2743, 87.1616) -> (-106.6843, 86.9917) projected
  line L280 (-106.6843, 86.9917) -> (-107.1243, 86.9338) projected
  line L281 (-107.1243, 86.9338) -> (-107.5643, 86.9917) projected
  line L282 (-107.5643, 86.9917) -> (-107.9743, 87.1615) projected
  line L283 (-107.9743, 87.1615) -> (-108.3264, 87.4317) projected
  line L284 (-108.3264, 87.4317) -> (-108.5965, 87.7838) projected
  line L285 (-108.5965, 87.7838) -> (-108.7664, 88.1938) projected
  line L286 (-37.6477, 33.6616) -> (-37.6729, 34.0619) projected
  line L287 (-37.6729, 34.0619) -> (-37.5977, 34.4559) projected
  line L288 (-37.5977, 34.4559) -> (-37.427, 34.8188) projected
  line L289 (-37.427, 34.8188) -> (-37.1713, 35.1278) projected
  line L290 (-37.1713, 35.1278) -> (-36.8469, 35.3636) projected
  line L291 (-36.8469, 35.3636) -> (-36.4739, 35.5112) projected
  line L292 (-36.4739, 35.5112) -> (-36.076, 35.5615) projected
  line L293 (-36.076, 35.5615) -> (-35.6781, 35.5112) projected
  line L294 (-35.6781, 35.5112) -> (-35.3052, 35.3636) projected
  line L295 (-35.3052, 35.3636) -> (-34.9808, 35.1278) projected
  line L296 (-34.9808, 35.1278) -> (-34.7251, 34.8188) projected
  line L297 (-34.7251, 34.8188) -> (-34.5543, 34.4559) projected
  line L298 (-34.5543, 34.4559) -> (-34.4792, 34.0619) projected
  line L299 (-34.4792, 34.0619) -> (-34.5044, 33.6616) projected
  line L300 (-34.5044, 33.6616) -> (-34.6283, 33.2802) projected
  line L301 (-34.6283, 33.2802) -> (-34.8432, 32.9416) projected
  line L302 (-34.8432, 32.9416) -> (-35.1356, 32.667) projected
  line L303 (-35.1356, 32.667) -> (-35.487, 32.4738) projected
  line L304 (-35.487, 32.4738) -> (-35.8755, 32.3741) projected
  line L305 (-35.8755, 32.3741) -> (-36.2766, 32.3741) projected
  line L306 (-36.2766, 32.3741) -> (-36.6651, 32.4738) projected
  line L307 (-36.6651, 32.4738) -> (-37.0165, 32.667) projected
  line L308 (-37.0165, 32.667) -> (-37.3089, 32.9416) projected
  line L309 (-37.3089, 32.9416) -> (-37.5238, 33.2802) projected
  line L310 (-37.5238, 33.2802) -> (-37.6477, 33.6616) projected
  line L311 (-149.2477, 33.6616) -> (-149.2729, 34.0619) projected
  line L312 (-149.2729, 34.0619) -> (-149.1977, 34.4559) projected
  line L313 (-149.1977, 34.4559) -> (-149.0269, 34.8188) projected
  line L314 (-149.0269, 34.8188) -> (-148.7713, 35.1278) projected
  line L315 (-148.7713, 35.1278) -> (-148.4468, 35.3636) projected
  line L316 (-148.4468, 35.3636) -> (-148.0739, 35.5112) projected
  line L317 (-148.0739, 35.5112) -> (-147.676, 35.5615) projected
  line L318 (-147.676, 35.5615) -> (-147.2781, 35.5112) projected
  line L319 (-147.2781, 35.5112) -> (-146.9052, 35.3635) projected
  line L320 (-146.9052, 35.3635) -> (-146.5807, 35.1278) projected
  line L321 (-146.5807, 35.1278) -> (-146.3251, 34.8188) projected
  line L322 (-146.3251, 34.8188) -> (-146.1543, 34.4559) projected
  line L323 (-146.1543, 34.4559) -> (-146.0792, 34.0619) projected
  line L324 (-146.0792, 34.0619) -> (-146.1044, 33.6616) projected
  line L325 (-146.1044, 33.6616) -> (-146.2283, 33.2802) projected
  line L326 (-146.2283, 33.2802) -> (-146.4432, 32.9416) projected
  line L327 (-146.4432, 32.9416) -> (-146.7356, 32.667) projected
  line L328 (-146.7356, 32.667) -> (-147.087, 32.4738) projected
  line L329 (-147.087, 32.4738) -> (-147.4755, 32.3741) projected
  line L330 (-147.4755, 32.3741) -> (-147.8766, 32.3741) projected
  line L331 (-147.8766, 32.3741) -> (-148.2651, 32.4738) projected
  line L332 (-148.2651, 32.4738) -> (-148.6165, 32.667) projected
  line L333 (-148.6165, 32.667) -> (-148.9088, 32.9416) projected
  line L334 (-148.9088, 32.9416) -> (-149.1238, 33.2802) projected
  line L335 (-149.1238, 33.2802) -> (-149.2477, 33.6616) projected
  line L336 (-19.376, 30.1615) -> (-19.376, 245.3788) projected
  line L337 (-19.376, 245.3788) -> (-25.876, 245.3788) projected
  line L338 (-25.876, 245.3788) -> (-25.876, 248.7288) projected
  line L339 (-25.876, 248.7288) -> (-31.8761, 248.7288) projected
  line L340 (-31.8761, 248.7288) -> (-31.8761, 245.3788) projected
  line L341 (-31.8761, 245.3788) -> (-37.9761, 245.3788) projected
  line L342 (-37.9761, 245.3788) -> (-37.9761, 239.3788) projected
  line L343 (-37.9761, 239.3788) -> (-36.7261, 239.3788) projected
  line L344 (-36.7261, 239.3788) -> (-36.7261, 237.3788) projected
  line L345 (-36.7261, 237.3788) -> (-37.9761, 237.3788) projected
  line L346 (-37.9761, 237.3788) -> (-37.9761, 234.7288) projected
  line L347 (-37.9761, 234.7288) -> (-40.9761, 234.7288) projected
  line L348 (-40.9761, 234.7288) -> (-40.9761, 237.3788) projected
  line L349 (-40.9761, 237.3788) -> (-42.226, 237.3788) projected
  line L350 (-42.226, 237.3788) -> (-42.226, 239.3788) projected
  line L351 (-42.226, 239.3788) -> (-40.9761, 239.3788) projected
  line L352 (-40.9761, 239.3788) -> (-40.9761, 245.3788) projected
  line L353 (-40.9761, 245.3788) -> (-47.0761, 245.3788) projected
  line L354 (-47.0761, 245.3788) -> (-47.0761, 248.7288) projected
  line L355 (-47.0761, 248.7288) -> (-53.076, 248.7288) projected
  line L356 (-53.076, 248.7288) -> (-53.076, 245.3788) projected
  line L357 (-53.076, 245.3788) -> (-134.0761, 245.3788) projected
  line L358 (-134.0761, 245.3788) -> (-134.0761, 248.7288) projected
  line L359 (-134.0761, 248.7288) -> (-140.0761, 248.7288) projected
  line L360 (-140.0761, 248.7288) -> (-140.0761, 245.3788) projected
  line L361 (-140.0761, 245.3788) -> (-146.176, 245.3788) projected
  line L362 (-146.176, 245.3788) -> (-146.176, 239.3788) projected
  line L363 (-146.176, 239.3788) -> (-144.926, 239.3788) projected
  line L364 (-144.926, 239.3788) -> (-144.926, 237.3788) projected
  line L365 (-144.926, 237.3788) -> (-146.176, 237.3788) projected
  line L366 (-146.176, 237.3788) -> (-146.176, 234.7288) projected
  line L367 (-146.176, 234.7288) -> (-149.1761, 234.7288) projected
  line L368 (-149.1761, 234.7288) -> (-149.1761, 237.3788) projected
  line L369 (-149.1761, 237.3788) -> (-150.4261, 237.3788) projected
  line L370 (-150.4261, 237.3788) -> (-150.4261, 239.3788) projected
  line L371 (-150.4261, 239.3788) -> (-149.1761, 239.3788) projected
  line L372 (-149.1761, 239.3788) -> (-149.1761, 245.3788) projected
  line L373 (-149.1761, 245.3788) -> (-155.2761, 245.3788) projected
  line L374 (-155.2761, 245.3788) -> (-155.2761, 248.7288) projected
  line L375 (-155.2761, 248.7288) -> (-161.276, 248.7288) projected
  line L376 (-161.276, 248.7288) -> (-161.276, 245.3788) projected
  line L377 (-161.276, 245.3788) -> (-196.376, 245.3788) projected
  line L378 (-196.376, 245.3788) -> (-196.376, 30.1615) projected
  line L379 (-196.376, 30.1615) -> (-19.376, 30.1615) projected
  circle A0 centre (-36.076, 33.9615) radius 1.5874
  circle A1 centre (-147.676, 33.9614) radius 1.5874
  circle A2 centre (-75.1211, 88.6342) radius 1.6855
  circle A3 centre (-107.1243, 88.6338) radius 1.6854
  circle A4 centre (-107.1228, 120.634) radius 1.6854
  circle A5 centre (-107.1236, 128.6339) radius 1.6854
  circle A6 centre (-75.1221, 120.634) radius 1.6855
  circle A7 centre (-75.1223, 128.634) radius 1.6855
  circle A8 centre (-75.1229, 160.6339) radius 1.6854
  circle A9 centre (-107.1228, 160.634) radius 1.6854
  point P0 (0, 0)
  constraints: 30 tangent, 10 centre point
hole "Hole1" at (-36.076, 3, -33.9615) at (-147.676, 3, -33.9614) at (-75.1211, 3, -88.6342) at (-107.1243, 3, -88.6338) at (-107.1228, 3, -120.634) at (-107.1236, 3, -128.6339) at (-75.1221, 3, -120.634) at (-75.1223, 3, -128.634) at (-75.1229, 3, -160.6339) at (-107.1228, 3, -160.634) direction (0, -1, 0) diameter 3.4 end through all
body "Solid1"
